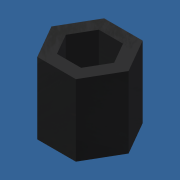
# Autodesk Inventor part: Nutspacker
Saved by Autodesk Inventor 2014 SP2 (Build 180246200, 246)
## iProperties
Created: 2015-02-01
Part Number: Nutspacker
Material: ABS-Kunststoff - Schwarz
Document SubType Name: Modeling
Designer: 4ndreas
Density: 1.06 g/cm^3
Appearance: Glatt - weiß(2)
Author: 4ndreas
Autodesk Inventor part; units mm, degrees
ref_plane "YZ Plane" through (0, 0, 0) normal (1, 0, 0) x (0, 1, 0)
sketch "Skizze1" plane through (0, 0, 0) normal (0, 0, 1) x (1, 0, 0)
  circle A0 centre (13.3363, -13.3273) radius 2.25 projected
  circle A1 centre (69.9048, -13.3273) radius 2.25 projected
  line L0 (49.1839, 14.957) -> (45.4022, 8.407) projected
  line L1 (45.4022, 8.407) -> (37.8389, 8.407) projected
  line L2 (37.8389, 8.407) -> (34.0573, 14.957) projected
  circle A2 centre (-86.3794, -2.543) radius 2.1 projected
  line L3 (-65.3794, -2.3212) -> (-80.3794, -2.3212) projected
  line L4 (-80.3794, -2.3212) -> (-80.3794, 8.457) projected
  line L5 (-80.3794, 8.457) -> (-86.3794, 8.457) projected
  line L6 (-86.3794, 8.457) -> (-86.3794, 3.857) projected
  line L7 (-86.3794, 3.857) -> (-93.3794, 3.857) projected
  line L8 (-93.3794, 3.857) -> (-93.3794, 8.457) projected
  line L9 (-93.3794, 8.457) -> (-98.3794, 8.457) projected
  line L10 (-98.3794, 8.457) -> (-98.3794, -15.043) projected
  line L11 (-38.3794, -15.043) -> (-98.3794, -15.043) projected
  spline S0 degree 3 poles (16.2456, -28.9938) (-0.41, -19.3777) (-19.1473, -15.043) (-38.3794, -15.043) knots 1 1 1 1 2 2 2 2 projected
  arc A3 (16.2456, -28.9938) -> (92.3706, 14.957) centre (41.6206, 14.957) ccw projected
  line L12 (-93.3794, 21.457) -> (-98.3794, 21.457) projected
  line L13 (-93.3794, 21.457) -> (-93.3794, 26.057) projected
  line L14 (-93.3794, 26.057) -> (-86.3794, 26.057) projected
  line L15 (-86.3794, 26.057) -> (-86.3794, 21.457) projected
  line L16 (-86.3794, 21.457) -> (-80.3794, 21.457) projected
  line L17 (-80.3794, 32.2352) -> (-80.3794, 21.457) projected
  line L18 (-65.3794, -4.043) -> (-65.3794, -2.3212) projected
  line L19 (26.6206, 28.1857) -> (26.6206, 1.7282) projected
  line L20 (26.6206, 1.7282) -> (16.7234, -4.043) projected
  line L21 (16.7234, -4.043) -> (-65.3794, -4.043) projected
  circle A4 centre (41.6206, 14.957) radius 4.1 construction
  line L22 (46.3548, 14.957) -> (43.9877, 19.057)
  line L23 (43.9877, 19.057) -> (39.2534, 19.057)
  line L24 (39.2534, 19.057) -> (36.8863, 14.957)
  line L25 (36.8863, 14.957) -> (39.2534, 10.857)
  line L26 (39.2534, 10.857) -> (43.9877, 10.857)
  line L27 (43.9877, 10.857) -> (46.3548, 14.957)
  arc A5 (92.3706, 14.957) -> (16.2456, 58.9078) centre (41.6206, 14.957) ccw projected
  spline S1 degree 3 poles (16.2456, 58.9078) (-0.41, 49.2917) (-19.1473, 44.957) (-38.3794, 44.957) knots 1 1 1 1 2 2 2 2 projected
  line L28 (-38.3794, 44.957) -> (-98.3794, 44.957) projected
  line L29 (-98.3794, 21.457) -> (-98.3794, 44.957) projected
  line L30 (-65.3794, 32.2352) -> (-80.3794, 32.2352) projected
  line L31 (-65.3794, 33.957) -> (-65.3794, 32.2352) projected
  line L32 (16.7234, 33.957) -> (-65.3794, 33.957) projected
  line L33 (26.6206, 28.1857) -> (16.7234, 33.957) projected
  circle A6 centre (13.3363, 43.2412) radius 2.25 projected
  circle A7 centre (69.9048, 43.2412) radius 2.25 projected
  circle A8 centre (-86.3794, 32.457) radius 2.1 projected
  line L34 (37.8389, 21.507) -> (34.0573, 14.957) projected
  line L35 (45.4022, 21.507) -> (37.8389, 21.507) projected
  line L36 (49.1839, 14.957) -> (45.4022, 21.507) projected
  point P0 (0, 0)
  dimension "d0" = 8.2
  constraints: 12 end point, 1 centre point, 1 tangent, 2 other
  measures "d0" diameter of A4
ref_plane "Arbeitsebene1" through (35.8206, 9.157, 7) normal (0, 0, -1) x (0, 1, 0)
ref_plane "Arbeitsebene2" through (35.8206, 9.157, -7) normal (0, 0, 1) x (1, 0, 0)
extrude "Extrusion1" add sketch "Skizze1" against normal up to surface (14 mm away) from surface at 7 contours L0 L1 L2 L34 L35 L36
